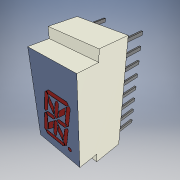
# Autodesk Inventor part: PSA39-21EWA
Saved by Autodesk Inventor 2018 (Build 220112000, 112)
## iProperties
Created: 2020-04-20
Part Number: PSA39-21EWA
Material: Všeobecné
Document SubType Name: Modeling
Designer: Jozko Mrkvicka
Density: 1 g/cm^3
Appearance: Výchozí
Author: Jozko Mrkvicka
Autodesk Inventor part; units mm, degrees
ref_plane "YZ Plane" through (0, 0, 0) normal (1, 0, 0) x (0, 1, 0)
ref_plane "XZ Plane" through (0, 0, 0) normal (0, 1, 0) x (-1, 0, 0)
ref_plane "XY Plane" through (0, 0, 0) normal (0, 0, 1) x (1, 0, 0)
sketch "Náčrt1" plane through (0, 0, 0) normal (0, 1, 0) x (-1, 0, 0)
  line L0 (0, 0) -> (20.955, 0)
  line L1 (20.955, 0) -> (20.955, -10.16)
  line L2 (20.955, -10.16) -> (0, -10.16)
  line L3 (0, -10.16) -> (0, 0)
  dimension "d0" = 20.955
  dimension "d1" = 10.16
  constraints: 8 end point, 2 parallel, 1 horizontal, 1 perpendicular
  measures "d0" distance of L1.end L2.end
  measures "d1" distance of L0.end L1.end
extrude "Vysunutí1" add sketch "Náčrt1" along normal blind 5.715
sketch "Náčrt3" plane through (0, 0, 0) normal (0, -1, 0) x (1, 0, 0)
  line L0 (-1.27, -1.4287) -> (-1.905, -1.4287)
  line L1 (-1.905, -1.4287) -> (-1.905, -1.1112)
  line L2 (-1.905, -1.1112) -> (-1.27, -1.1112)
  line L3 (-1.27, -1.1112) -> (-1.27, -1.4287)
  line L4 (-3.81, -1.4287) -> (-4.445, -1.4287)
  line L5 (-4.445, -1.4287) -> (-4.445, -1.1112)
  line L6 (-4.445, -1.1112) -> (-3.81, -1.1112)
  line L7 (-3.81, -1.1112) -> (-3.81, -1.4287)
  line L8 (-6.35, -1.4287) -> (-6.985, -1.4288)
  line L9 (-6.985, -1.4288) -> (-6.985, -1.1112)
  line L10 (-6.985, -1.1112) -> (-6.35, -1.1112)
  line L11 (-6.35, -1.1112) -> (-6.35, -1.4287)
  line L12 (-8.89, -1.4287) -> (-9.525, -1.4287)
  line L13 (-9.525, -1.4287) -> (-9.525, -1.1112)
  line L14 (-9.525, -1.1112) -> (-8.89, -1.1112)
  line L15 (-8.89, -1.1112) -> (-8.89, -1.4287)
  line L16 (-11.43, -1.4287) -> (-12.065, -1.4287)
  line L17 (-12.065, -1.4287) -> (-12.065, -1.1112)
  line L18 (-12.065, -1.1112) -> (-11.43, -1.1112)
  line L19 (-11.43, -1.1112) -> (-11.43, -1.4287)
  line L20 (-12.065, -8.7313) -> (-11.43, -8.7313)
  line L21 (-11.43, -8.7313) -> (-11.43, -9.0488)
  line L22 (-11.43, -9.0488) -> (-12.065, -9.0488)
  line L23 (-12.065, -9.0488) -> (-12.065, -8.7313)
  line L24 (-9.525, -8.7313) -> (-8.89, -8.7313)
  line L25 (-8.89, -8.7313) -> (-8.89, -9.0488)
  line L26 (-8.89, -9.0488) -> (-9.525, -9.0488)
  line L27 (-9.525, -9.0488) -> (-9.525, -8.7313)
  line L28 (-6.985, -8.7313) -> (-6.35, -8.7313)
  line L29 (-6.35, -8.7313) -> (-6.35, -9.0487)
  line L30 (-6.35, -9.0487) -> (-6.985, -9.0488)
  line L31 (-6.985, -9.0488) -> (-6.985, -8.7313)
  line L32 (-4.445, -8.7313) -> (-3.81, -8.7313)
  line L33 (-3.81, -8.7313) -> (-3.81, -9.0487)
  line L34 (-3.81, -9.0487) -> (-4.445, -9.0488)
  line L35 (-4.445, -9.0488) -> (-4.445, -8.7313)
  line L36 (-1.905, -8.7313) -> (-1.27, -8.7312)
  line L37 (-1.27, -8.7312) -> (-1.27, -9.0487)
  line L38 (-1.27, -9.0487) -> (-1.905, -9.0488)
  line L39 (-1.905, -9.0488) -> (-1.905, -8.7313)
  line L40 (-13.97, -1.4287) -> (-14.605, -1.4287)
  line L41 (-14.605, -1.4287) -> (-14.605, -1.1112)
  line L42 (-14.605, -1.1112) -> (-13.97, -1.1112)
  line L43 (-13.97, -1.1112) -> (-13.97, -1.4287)
  line L44 (-14.605, -8.7313) -> (-13.97, -8.7313)
  line L45 (-13.97, -8.7313) -> (-13.97, -9.0488)
  line L46 (-13.97, -9.0488) -> (-14.605, -9.0488)
  line L47 (-14.605, -9.0488) -> (-14.605, -8.7313)
  line L48 (-16.51, -1.4288) -> (-17.145, -1.4288)
  line L49 (-17.145, -1.4288) -> (-17.145, -1.1113)
  line L50 (-17.145, -1.1113) -> (-16.51, -1.1113)
  line L51 (-16.51, -1.1113) -> (-16.51, -1.4288)
  line L52 (-17.145, -8.7313) -> (-16.51, -8.7313)
  line L53 (-16.51, -8.7313) -> (-16.51, -9.0488)
  line L54 (-16.51, -9.0488) -> (-17.145, -9.0488)
  line L55 (-17.145, -9.0488) -> (-17.145, -8.7313)
  line L56 (-19.05, -1.4287) -> (-19.685, -1.4287)
  line L57 (-19.685, -1.4287) -> (-19.685, -1.1112)
  line L58 (-19.685, -1.1112) -> (-19.05, -1.1112)
  line L59 (-19.05, -1.1112) -> (-19.05, -1.4287)
  line L60 (-19.685, -8.7313) -> (-19.05, -8.7313)
  line L61 (-19.05, -8.7313) -> (-19.05, -9.0488)
  line L62 (-19.05, -9.0488) -> (-19.685, -9.0488)
  line L63 (-19.685, -9.0488) -> (-19.685, -8.7313)
  point P0 (-6.6675, -1.27)
  point P1 (-6.6675, -8.89)
  point P2 (-4.1275, -1.27)
  point P3 (-9.2075, -1.27)
  point P4 (-4.1275, -8.89)
  point P5 (-9.2075, -8.89)
  point P6 (-1.5875, -1.27)
  point P7 (-4.1275, -1.27)
  point P8 (-6.6675, -1.27)
  point P9 (-9.2075, -1.27)
  point P10 (-11.7475, -1.27)
  point P11 (-11.7475, -8.89)
  point P12 (-9.2075, -8.89)
  point P13 (-6.6675, -8.89)
  point P14 (-4.1275, -8.89)
  point P15 (-1.5875, -8.89)
  point P16 (-14.2875, -1.27)
  point P17 (-14.2875, -8.89)
  point P18 (-16.8275, -1.27)
  point P19 (-16.8275, -8.89)
  point P20 (-19.3675, -1.27)
  point P21 (-19.3675, -8.89)
  point P22 (-1.5875, -1.27)
  point P23 (-1.5875, -8.89)
  constraints: 128 end point, 32 parallel, 16 perpendicular
sketch "Náčrt4" plane through (0, 0, 0) normal (0, -1, 0) x (1, 0, 0)
  line L0 (-3.81, -8.7313) -> (-3.81, -9.0487) projected
  line L1 (-3.81, -9.0487) -> (-4.445, -9.0488) projected
  line L2 (-4.445, -9.0488) -> (-4.445, -8.7313) projected
  line L3 (-4.445, -8.7313) -> (-3.81, -8.7313) projected
  line L4 (-8.89, -8.7313) -> (-8.89, -9.0488) projected
  line L5 (-8.89, -9.0488) -> (-9.525, -9.0488) projected
  line L6 (-9.525, -9.0488) -> (-9.525, -8.7313) projected
  line L7 (-9.525, -8.7313) -> (-8.89, -8.7313) projected
  line L8 (-12.065, -1.4287) -> (-12.065, -1.1112) projected
  line L9 (-12.065, -1.1112) -> (-11.43, -1.1112) projected
  line L10 (-11.43, -1.1112) -> (-11.43, -1.4287) projected
  line L11 (-11.43, -1.4287) -> (-12.065, -1.4287) projected
  line L12 (-6.985, -1.4288) -> (-6.985, -1.1112) projected
  line L13 (-6.985, -1.1112) -> (-6.35, -1.1112) projected
  line L14 (-6.35, -1.1112) -> (-6.35, -1.4287) projected
  line L15 (-6.35, -1.4287) -> (-6.985, -1.4288) projected
  line L16 (-1.905, -1.4287) -> (-1.905, -1.1112) projected
  line L17 (-1.905, -1.1112) -> (-1.27, -1.1112) projected
  line L18 (-1.27, -1.1112) -> (-1.27, -1.4287) projected
  line L19 (-1.27, -1.4287) -> (-1.905, -1.4287) projected
  line L20 (-4.445, -1.4287) -> (-4.445, -1.1112) projected
  line L21 (-4.445, -1.1112) -> (-3.81, -1.1112) projected
  line L22 (-3.81, -1.1112) -> (-3.81, -1.4287) projected
  line L23 (-3.81, -1.4287) -> (-4.445, -1.4287) projected
  line L24 (-9.525, -1.4287) -> (-9.525, -1.1112) projected
  line L25 (-9.525, -1.1112) -> (-8.89, -1.1112) projected
  line L26 (-8.89, -1.1112) -> (-8.89, -1.4287) projected
  line L27 (-8.89, -1.4287) -> (-9.525, -1.4287) projected
  line L28 (-11.43, -8.7313) -> (-11.43, -9.0488) projected
  line L29 (-11.43, -9.0488) -> (-12.065, -9.0488) projected
  line L30 (-12.065, -9.0488) -> (-12.065, -8.7313) projected
  line L31 (-12.065, -8.7313) -> (-11.43, -8.7313) projected
  line L32 (-6.35, -8.7313) -> (-6.35, -9.0487) projected
  line L33 (-6.35, -9.0487) -> (-6.985, -9.0488) projected
  line L34 (-6.985, -9.0488) -> (-6.985, -8.7313) projected
  line L35 (-6.985, -8.7313) -> (-6.35, -8.7313) projected
  line L36 (-1.27, -8.7312) -> (-1.27, -9.0487) projected
  line L37 (-1.27, -9.0487) -> (-1.905, -9.0488) projected
  line L38 (-1.905, -9.0488) -> (-1.905, -8.7313) projected
  line L39 (-1.905, -8.7313) -> (-1.27, -8.7312) projected
  line L40 (-0.3175, -1.5968) -> (-0.3175, -0.3175)
  line L41 (-0.3175, -9.8173) -> (-0.3175, -1.5968)
  line L42 (-20.6375, -2.8575) -> (-20.6375, -9.8425)
  line L43 (-0.3175, -9.8173) -> (-20.6375, -9.8425)
  line L44 (-1.5968, -0.3175) -> (-0.3175, -0.3175)
  line L45 (-20.955, -10.16) -> (-20.32, -10.16)
  line L46 (-1.5968, -0.3175) -> (-20.6375, -0.3175)
  line L47 (-20.6375, -2.8575) -> (-20.6375, -0.3175)
  line L48 (-13.97, -1.1112) -> (-14.605, -1.1112)
  line L49 (-14.605, -1.1112) -> (-14.605, -1.4287)
  line L50 (-14.605, -1.4287) -> (-13.97, -1.4287)
  line L51 (-13.97, -1.4287) -> (-13.97, -1.1112)
  line L52 (-16.51, -1.1112) -> (-17.145, -1.1112)
  line L53 (-17.145, -1.1112) -> (-17.145, -1.4287)
  line L54 (-17.145, -1.4287) -> (-16.51, -1.4287)
  line L55 (-16.51, -1.4287) -> (-16.51, -1.1112)
  line L56 (-19.05, -1.1112) -> (-19.685, -1.1112)
  line L57 (-19.685, -1.1112) -> (-19.685, -1.4287)
  line L58 (-19.685, -1.4287) -> (-19.05, -1.4287)
  line L59 (-19.05, -1.4287) -> (-19.05, -1.1112)
  line L60 (-13.97, -8.7313) -> (-14.605, -8.7313)
  line L61 (-14.605, -8.7313) -> (-14.605, -9.0488)
  line L62 (-14.605, -9.0488) -> (-13.97, -9.0488)
  line L63 (-13.97, -9.0488) -> (-13.97, -8.7313)
  line L64 (-16.51, -8.7313) -> (-17.145, -8.7313)
  line L65 (-17.145, -8.7313) -> (-17.145, -9.0488)
  line L66 (-17.145, -9.0488) -> (-16.51, -9.0488)
  line L67 (-16.51, -9.0488) -> (-16.51, -8.7313)
  line L68 (-19.05, -8.7313) -> (-19.685, -8.7313)
  line L69 (-19.685, -8.7313) -> (-19.685, -9.0488)
  line L70 (-19.685, -9.0488) -> (-19.05, -9.0488)
  line L71 (-19.05, -9.0488) -> (-19.05, -8.7313)
  point P0 (-8.5818, -2.8575)
  point P1 (-20.6375, -9.8425)
  constraints: 64 end point, 14 point on line, 12 parallel, 8 horizontal, 6 perpendicular, 3 vertical
extrude "Vysunutí4" cut sketch "Náčrt4" against normal blind 1.27 contours L41 L43 L42 L47 L46 L44 L40 | L51 L50 L49 L48 | L55 L54 L53 L52 | L59 L58 L57 L56 | L63 L62 L61 L60 | L67 L66 L65 L64 | L71 L70 L69 L68
extrude "Vysunutí7" add sketch "Náčrt3" along normal blind 5.08
sketch "Náčrt7" plane through (0, 1.27, 0) normal (0, -1, 0) x (1, 0, 0)
  line L0 (-13.97, -1.1112) -> (-14.605, -1.1112) projected
  line L1 (-13.97, -1.4287) -> (-13.97, -1.1112) projected
  line L2 (-14.605, -1.4287) -> (-13.97, -1.4287) projected
  line L3 (-14.605, -1.1112) -> (-14.605, -1.4287) projected
  line L4 (-17.145, -1.4288) -> (-16.51, -1.4288) projected
  line L5 (-17.145, -1.1113) -> (-17.145, -1.4288) projected
  line L6 (-16.51, -1.1113) -> (-17.145, -1.1113) projected
  line L7 (-17.145, -1.4288) -> (-16.51, -1.4288) projected
  line L8 (-16.51, -1.4288) -> (-16.51, -1.1113) projected
  line L9 (-16.51, -1.1113) -> (-17.145, -1.1113) projected
  line L10 (-17.145, -1.1113) -> (-17.145, -1.4288) projected
  line L11 (-19.685, -1.4287) -> (-19.05, -1.4287) projected
  line L12 (-19.05, -1.4287) -> (-19.05, -1.1112) projected
  line L13 (-19.05, -1.1112) -> (-19.685, -1.1112) projected
  line L14 (-19.685, -1.1112) -> (-19.685, -1.4287) projected
  line L15 (-19.05, -8.7313) -> (-19.685, -8.7313) projected
  line L16 (-19.685, -8.7313) -> (-19.685, -9.0488) projected
  line L17 (-19.685, -9.0488) -> (-19.05, -9.0488) projected
  line L18 (-19.05, -9.0488) -> (-19.05, -8.7313) projected
  line L19 (-16.51, -8.7313) -> (-17.145, -8.7313) projected
  line L20 (-17.145, -8.7313) -> (-17.145, -9.0488) projected
  line L21 (-17.145, -9.0488) -> (-16.51, -9.0488) projected
  line L22 (-16.51, -9.0488) -> (-16.51, -8.7313) projected
  line L23 (-13.97, -8.7313) -> (-14.605, -8.7313) projected
  line L24 (-14.605, -8.7313) -> (-14.605, -9.0488) projected
  line L25 (-14.605, -9.0488) -> (-13.97, -9.0488) projected
  line L26 (-13.97, -9.0488) -> (-13.97, -8.7313) projected
  point P0 (0, 0)
extrude "Vysunutí8" add sketch "Náčrt7" along normal up to surface (1.27 mm away)
sketch "Náčrt9" plane through (0, 5.715, 0) normal (0, 1, 0) x (1, 0, 0)
  line L0 (-1.905, 10.16) -> (-19.05, 10.16)
  line L1 (-19.05, 10.16) -> (-19.05, 0)
  line L2 (-19.05, 0) -> (-1.905, 0)
  line L3 (-1.905, 0) -> (-1.905, 10.16)
  constraints: 8 end point, 2 parallel, 1 horizontal, 1 perpendicular
extrude "Vysunutí10" add sketch "Náčrt9" along normal blind 3.81
sketch "Náčrt10" plane through (0, 9.525, 0) normal (0, 1, 0) x (1, 0, 0)
  line L0 (-8.2122, 2.3686) -> (-8.2314, 6.4318)
  line L1 (-8.4126, 2.4039) -> (-7.9019, 1.8137)
  line L2 (-7.9019, 1.8137) -> (-8.2067, 1.5598)
  line L3 (-7.8036, 1.8964) -> (-8.2122, 2.3686)
  line L4 (-7.3989, 6.3003) -> (-7.3989, 2.237)
  line L5 (-7.3989, 2.237) -> (-7.8036, 1.8964)
  line L6 (-7.8267, 6.7723) -> (-7.3989, 6.3003)
  line L7 (-7.8267, 6.7723) -> (-8.2314, 6.4318)
  line L8 (-8.4098, 6.4696) -> (-7.9006, 6.898)
  line L9 (-8.4098, 6.4696) -> (-11.4573, 6.9775)
  line L10 (-7.9006, 6.898) -> (-8.1935, 7.2462)
  line L11 (-8.1935, 7.2462) -> (-11.8636, 7.8578)
  line L12 (-8.4126, 2.4039) -> (-11.5949, 2.9187)
  line L13 (-11.8636, 2.1693) -> (-8.2067, 1.5598)
  line L14 (-11.5949, 2.9187) -> (-12.118, 2.466)
  line L15 (-12.118, 2.466) -> (-11.8636, 2.1693)
  line L16 (-11.8636, 2.9819) -> (-12.2699, 2.6433)
  line L17 (-16.3332, 3.7268) -> (-16.3332, 7.7901)
  line L18 (-17.1459, 3.8623) -> (-17.1459, 7.9256)
  line L19 (-12.9471, 7.2258) -> (-16.1301, 7.7563)
  line L20 (-17.1459, 7.9256) -> (-16.7395, 8.2642)
  line L21 (-16.3332, 7.7901) -> (-16.7395, 8.2642)
  line L22 (-16.1301, 7.7563) -> (-16.638, 8.3488)
  line L23 (-16.638, 8.3488) -> (-16.3332, 8.6028)
  line L24 (-12.6763, 7.9933) -> (-16.3332, 8.6028)
  line L25 (-12.4032, 7.6791) -> (-12.6763, 7.9933)
  line L26 (-12.9471, 7.2258) -> (-12.4032, 7.6791)
  line L27 (-12.2699, 7.5192) -> (-12.6763, 7.1806)
  line L28 (-12.0842, 7.674) -> (-11.4573, 6.9775)
  line L29 (-11.8636, 7.0452) -> (-12.2699, 7.5192)
  line L30 (-12.0842, 7.674) -> (-11.8636, 7.8578)
  line L31 (-12.2699, 2.6433) -> (-12.6763, 3.1174)
  line L32 (-13.0826, 3.1851) -> (-12.4534, 2.486)
  line L33 (-12.4534, 2.486) -> (-12.6763, 2.3047)
  line L34 (-13.0826, 3.1851) -> (-16.1253, 3.6922)
  line L35 (-16.3332, 3.7268) -> (-16.7395, 3.3882)
  line L36 (-16.1253, 3.6922) -> (-16.6296, 3.26)
  line L37 (-16.7395, 3.3882) -> (-17.1459, 3.8623)
  line L38 (-16.6296, 3.26) -> (-16.3332, 2.9142)
  circle A0 centre (-16.7395, 2.237) radius 0.4063
  line L39 (-16.3332, 2.9142) -> (-12.6763, 2.3047)
  line L40 (-11.8636, 5.649) -> (-12.2774, 5.3042)
  line L41 (-12.2774, 5.3042) -> (-12.6763, 5.7695)
  line L42 (-11.8636, 4.356) -> (-12.2737, 4.8345)
  line L43 (-12.2724, 4.8356) -> (-12.6763, 4.499)
  line L44 (-12.0842, 5.0499) -> (-11.7075, 4.6104)
  line L45 (-12.0842, 5.0499) -> (-11.6884, 5.3797)
  line L46 (-12.4731, 5.1147) -> (-12.869, 5.5766)
  line L47 (-12.4731, 5.1147) -> (-12.8497, 4.8009)
  line L48 (-11.8636, 4.356) -> (-11.8636, 2.9819)
  line L49 (-12.2724, 4.8356) -> (-12.2724, 4.8329)
  line L50 (-12.6763, 3.1174) -> (-12.6763, 4.499)
  line L51 (-12.6763, 5.7695) -> (-12.6763, 7.1806)
  line L52 (-11.8636, 7.0452) -> (-11.8636, 5.649)
  line L53 (-8.4126, 4.4377) -> (-8.7893, 4.1238)
  line L54 (-8.4126, 4.4377) -> (-8.8085, 4.8995)
  line L55 (-16.1366, 5.7256) -> (-15.7408, 6.0555)
  line L56 (-16.1366, 5.7256) -> (-15.7599, 5.2861)
  line L57 (-8.8085, 4.8995) -> (-11.6884, 5.3797)
  line L58 (-8.7893, 4.1238) -> (-11.7075, 4.6104)
  line L59 (-12.869, 5.5766) -> (-15.7408, 6.0555)
  line L60 (-12.8497, 4.8009) -> (-15.7599, 5.2861)
  line L61 (-11.552, 5.543) -> (-10.0136, 6.5477)
  line L62 (-8.5737, 6.3077) -> (-10.112, 5.303)
  line L63 (-13.0357, 4.6459) -> (-14.5126, 3.6094)
  line L64 (-15.9437, 3.8479) -> (-14.4668, 4.8844)
  line L65 (-13.0549, 5.7935) -> (-14.316, 7.2648)
  line L66 (-15.9409, 7.5356) -> (-14.6798, 6.0643)
  line L67 (-8.5737, 6.3077) -> (-10.0136, 6.5477)
  line L68 (-10.112, 5.303) -> (-11.552, 5.543)
  line L69 (-10.112, 4.1586) -> (-11.5216, 4.3935)
  line L70 (-8.8085, 2.6587) -> (-10.0105, 2.859)
  line L71 (-13.0549, 5.7935) -> (-14.6798, 6.0643)
  line L72 (-13.0357, 4.6459) -> (-14.4668, 4.8844)
  line L73 (-14.5126, 3.6094) -> (-15.9437, 3.8479)
  line L74 (-14.316, 7.2648) -> (-15.9409, 7.5356)
  line L75 (-10.112, 4.1586) -> (-8.6009, 2.6241)
  line L76 (-11.5216, 4.3935) -> (-10.0105, 2.859)
  line L77 (-8.8085, 2.6587) -> (-8.6009, 2.6241)
  point P0 (0, 0)
  point P1 (-7.3989, 6.3003)
  point P2 (-6.5813, 1.018)
  point P3 (-6.5813, 9.1446)
  point P4 (-17.9585, 9.1446)
  point P5 (-17.9585, 1.018)
  point P6 (-16.3332, 5.7585)
  point P7 (-17.1459, 5.8939)
  point P8 (-7.3989, 4.2686)
  constraints: 156 end point, 39 parallel, 15 point on line, 3 midpoint, 3 perpendicular, 1 centre point, 1 vertical
extrude "Vysunutí11" cut sketch "Náčrt10" against normal blind 0.0254
